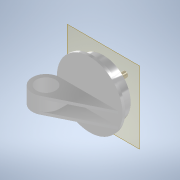
# Autodesk Inventor part: C1
Saved by Autodesk Inventor 2022.2 (Build 262287010, 287A)
## iProperties
Created: 2022-04-10
Part Number: C1
Material: Aluminum 6061
Document SubType Name: Modeling
Designer: stasi
Density: 2.7 g/cm^3
Appearance: Aluminum - Flat
Mass: 723.228 g
Surface Area: 475.401 cm^2
Volume: 267.862 cm^3
Author: stasi
Autodesk Inventor part; units mm, degrees
ref_plane "YZ Plane" through (0, 0, 0) normal (1, 0, 0) x (0, 1, 0)
ref_plane "XZ Plane" through (0, 0, 0) normal (0, 1, 0) x (-1, 0, 0)
ref_plane "XY Plane" through (0, 0, 0) normal (0, 0, 1) x (1, 0, 0)
ref_plane "Work Plane2" through (0, 0, 0) normal (0, 0, 1) x (1, 0, 0)
sketch "Sketch2" plane through (0, 0, 0) normal (0, 0, 1) x (1, 0, 0)
  circle A0 centre (0, 0) radius 60
  dimension "d0" = 120
  constraints: 1 centre point, 1 coincident
  measures "d0" diameter of A0
extrude "podstawa c1" add sketch "Sketch2" along normal blind 25
sketch "Sketch9" plane through (0, 0, 0) normal (0, 0, -1) x (-1, 0, 0)
  line L0 (0, 0) -> (0, -30) projected
  circle A0 centre (0, 0) radius 5
  dimension "d18" = 10
  constraints: 1 centre point, 1 coincident
  measures "d18" diameter of A0
extrude "wal c1" add sketch "Sketch9" along normal blind 40
sketch "Sketch11" plane through (0, 0, 25) normal (0, 0, 1) x (1, 0, 0)
  circle A0 centre (0, 0) radius 5 projected
  circle A1 centre (0, 0) radius 60 projected
  line L0 (0, 0) -> (51.9615, 0)
  line L1 (51.9615, 0) -> (51.9615, -30)
  line L2 (51.9615, -30) -> (0, -30)
  line L3 (0, -30) -> (0, 0)
  line L4 (0, 0) -> (-80, 0)
  line L5 (-80, 0) -> (-80, -30)
  line L6 (-80, -30) -> (0, -30)
  line L7 (0, -30) -> (0, 0)
  line L8 (51.9615, 0) -> (-80, 0)
  line L9 (-80, 0) -> (-80, -30)
  line L10 (-80, -30) -> (51.9615, -30)
  line L11 (51.9615, -30) -> (51.9615, 0)
  dimension "d23" = 30
  dimension "d24" = 80
  dimension "d47" = 51.9615
  dimension "d48" = 30
  constraints: 24 end point, 6 parallel, 3 horizontal, 3 perpendicular, 1 point on line, 2 other
  measures "d23" distance of L0.end L1.end
  measures "d24" distance of L6.end L5.end
  measures "d47" distance from line of point (0, -30) L1
  measures "d48" distance from line of point (0, -30) L8
extrude "mocowanie c2" add sketch "Sketch11" along normal blind 50 contours L0 L1 L2 L3 A0 | A0 L3 L0 | L4 L3 A0 | A0 L3 L6 A1 L4 | A1 L6 L5 L4
sketch "Sketch12" plane through (-80, 0, 25) normal (0, 1, 0) x (1, 0, 0)
  line L0 (20, 0) -> (0, 0) projected
  line L1 (131.9615, -50) -> (0, -50) projected
  line L2 (0, 0) -> (131.9615, 0)
  line L3 (131.9615, 0) -> (131.9615, -50)
  line L4 (131.9615, -50) -> (0, -50)
  line L5 (0, -50) -> (0, 0)
  line L6 (0, 0) -> (80, 0)
  line L7 (80, 0) -> (80, -50)
  line L8 (80, -50) -> (0, -50)
  line L9 (0, -50) -> (0, 0)
  circle A0 centre (25, -25) radius 17.5
  point P0 (80, 25)
  dimension "d27" = 80
  dimension "d28" = 50
  dimension "d30" = 35
  dimension "d49" = 25
  dimension "d50" = 106.9615
  constraints: 16 end point, 4 parallel, 2 horizontal, 2 perpendicular, 1 centre point, 1 point on line
  measures "d27" distance of L7.end L8.end
  measures "d28" distance of L2.end L1.start
  measures "d30" diameter of A0
  measures "d49" distance from line of A0.centre L1
  measures "d50" distance from line of A0.centre L3
extrude "wneka na wal c2" cut sketch "Sketch12" against normal blind 30 contours A0
full round fillet "Full Round Fillet1" first side at (-36.0128, -10, 75) centre faces at (-80, -10, 41.6667) second side at (-73.0295, -13.473, 25)
sketch "Sketch14" plane through (-60, 0, 25) normal (0, 1, 0) x (1, 0, 0)
  circle A0 centre (5, -25) radius 5 projected
  circle A1 centre (5, -25) radius 25
  line L0 (8.0385, 0) -> (111.9615, 0) projected
  line L1 (111.9615, 0) -> (16.0811, -47.41)
  line L2 (111.9615, 0) -> (111.9615, -50) projected
  line L3 (111.9615, -50) -> (111.9615, 0)
  line L4 (16.0811, -47.41) -> (111.9615, -47.41)
  point P0 (60, 25)
  constraints: 6 end point, 1 coincident, 1 collinear, 1 perpendicular, 1 point on line, 4 other
extrude "odchudzenie 1" cut sketch "Sketch14" against normal blind 30 contours L1 L2 L4
sketch "Sketch15" plane through (51.9615, 0, 72.41) normal (0, 0, -1) x (-1, 0, 0)
  line L0 (106.9615, -30) -> (0, -30) projected
  line L1 (95.8804, 0) -> (95.8804, -30) projected
  line L2 (95.8804, -30) -> (95.8804, 0)
  line L3 (0, -30) -> (0, 0) projected
  line L4 (95.8804, 0) -> (0, 0)
  line L5 (0, 0) -> (0, -30)
  line L6 (0, -30) -> (95.8804, -30)
  point P0 (51.9615, 0)
  constraints: 8 end point, 3 perpendicular, 1 collinear, 1 point on line
extrude "odchudzenie 2" cut sketch "Sketch15" against normal blind 30
sketch "Sketch16" plane through (-60, 0, 25) normal (0, 1, 0) x (1, 0, 0)
  circle A0 centre (5, -25) radius 5 projected
  circle A1 centre (5, -25) radius 25
  line L0 (111.9615, 0) -> (16.0811, -47.41) projected
  line L1 (16.0811, -50) -> (16.0811, -47.41) projected
  line L2 (16.0811, -47.41) -> (16.0811, -50)
  line L3 (5, -50) -> (16.0811, -50) projected
  line L4 (16.0811, -50) -> (5, -50)
  point P0 (60, 25)
  constraints: 4 end point, 1 centre point, 1 coincident, 1 collinear, 1 perpendicular, 1 tangent
extrude "odchudznie 3" cut sketch "Sketch16" against normal blind 30 contours A1 L1 L3
sketch "Sketch17" plane through (-60, 0, 25) normal (0, 1, 0) x (1, 0, 0)
  point P0 (60, 25)
sketch "Sketch18" plane through (0, 0, 25) normal (0, 0, 1) x (1, 0, 0)
  line L0 (51.9615, 0) -> (51.9615, -30) projected
  line L1 (51.9615, -5) -> (-29.9985, -5)
  line L2 (-29.9985, -5) -> (-29.9985, -25)
  line L3 (-29.9985, -25) -> (51.9615, -25)
  line L4 (51.9615, -25) -> (51.9615, -5)
  point P0 (0, 0)
  dimension "d42" = 81.96
  dimension "d43" = 20
  dimension "d52" = 5
  dimension "d53" = 0
  dimension "d54" = 20
  constraints: 8 end point, 2 parallel, 1 horizontal, 1 perpendicular, 1 point on line
  measures "d42" distance of L3.end L2.end
  measures "d43" distance of L2.end L1.end
  measures "d52" distance from line of L0.start L1
  measures "d53" distance from line of point (51.962, -25) L0
  measures "d54" distance from line of point (51.962, -25) L1
extrude "odchudzenie 4" cut sketch "Sketch18" along normal blind 50
fillet "Fillet3" radius 25 1 edges at (-29.9985, -15, 65.5268)
sketch "Sketch20" plane through (0, 0, 0) normal (0, 0, -1) x (-1, 0, 0)
  circle A0 centre (0, 0) radius 50
  circle A1 centre (0, 0) radius 60
  dimension "d55" = 100
  constraints: 2 centre point, 2 coincident
  measures "d55" diameter of A0
extrude "wyciecie dla łożyska c0" cut sketch "Sketch20" against normal blind 20
body "Solid1"
